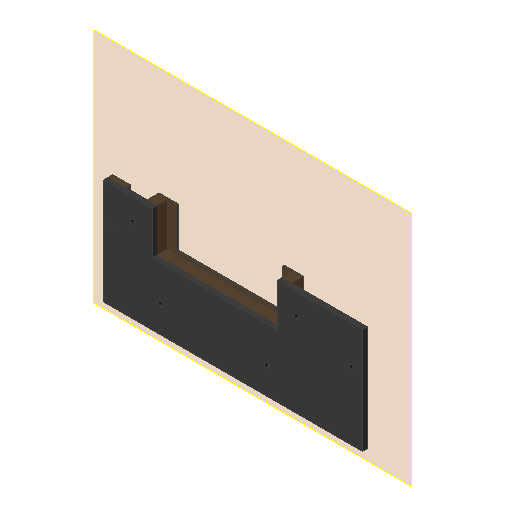
# Autodesk Inventor part: 30_XYTabel_Aliexpress_cellSTORM_chiptray
Saved by Autodesk Inventor 2022 (Build 260153000, 153)
## iProperties
Created: 2021-12-30
Part Number: 30_XYTabel_Aliexpress_cellSTORM_chiptray
Material: Generisch
Document SubType Name: Modeling
Designer: diederichbenedict
Density: 1 g/cm^3
Appearance: Vorgabe
Author: diederichbenedict
Autodesk Inventor part; units mm, degrees
ref_plane "YZ Plane" through (0, 0, 0) normal (1, 0, 0) x (0, 1, 0)
ref_plane "Arbeitsebene1" through (0, 0, 0) normal (0, 0, 1) x (1, 0, 0)
sketch "Skizze1" plane through (0, 0, 0) normal (0, 0, 1) x (1, 0, 0)
  circle A0 centre (-54.34, -50.59) radius 1.5 projected
  circle A1 centre (11.66, -50.59) radius 1.5 projected
  circle A2 centre (-85.34, -22.83) radius 1 projected
  circle A3 centre (-85.34, -22.83) radius 1 construction
  circle A4 centre (-85.34, 37.77) radius 1 construction
  line L0 (37.14, -42.13) -> (37.14, -36.73) construction
  arc A5 (32.14, -41.73) -> (37.14, -36.73) centre (32.14, -36.73) ccw construction
  line L1 (32.14, -41.73) -> (-73.22, -41.73) construction
  arc A6 (-78.22, -36.73) -> (-73.22, -41.73) centre (-73.22, -36.73) ccw construction
  line L2 (-78.22, -36.73) -> (-78.22, 48.27) construction
  arc A7 (-73.22, 53.27) -> (-78.22, 48.27) centre (-73.22, 48.27) ccw construction
  line L3 (-73.22, 53.27) -> (32.14, 53.27) construction
  arc A8 (37.14, 48.27) -> (32.14, 53.27) centre (32.14, 48.27) ccw construction
  line L4 (37.14, 48.27) -> (37.14, 54.21) construction
  line L5 (37.14, 54.21) -> (-89.84, 54.21) construction
  line L6 (-89.84, 54.21) -> (-89.84, -42.13) construction
  line L7 (-89.84, -42.13) -> (37.14, -42.13) construction
  circle A9 centre (64.84, -24.91) radius 1.5 construction
  circle A10 centre (-85.34, -43.41) radius 1 construction
  circle A11 centre (64.84, 35.59) radius 1.5 construction
  circle A12 centre (11.66, -50.59) radius 1.5 construction
  circle A13 centre (-54.34, -50.59) radius 1.5 construction
  circle A14 centre (-85.34, 58.59) radius 1 construction
  line L8 (-89.84, 67.09) -> (-89.84, 54.21) construction
  line L9 (-89.84, 54.21) -> (37.14, 54.21) construction
  line L10 (37.14, 54.21) -> (37.14, -42.13) construction
  line L11 (37.14, -42.13) -> (-89.84, -42.13) construction
  line L12 (-89.84, -42.13) -> (-89.84, -67.09) construction
  line L13 (-89.84, -67.09) -> (89.84, -67.09) construction
  line L14 (89.84, -67.09) -> (89.84, 67.09) construction
  line L15 (89.84, 67.09) -> (-89.84, 67.09) construction
  line L16 (-58.54, -1.33) -> (17.46, -1.33) construction
  line L17 (-58.54, -27.13) -> (-58.54, -1.33) construction
  line L18 (17.46, -27.13) -> (-58.54, -27.13) construction
  line L19 (17.46, -1.33) -> (17.46, -27.13) construction
  line L20 (-89.84, -1.33) -> (-59.54, -1.33)
  line L21 (-59.54, -1.33) -> (-59.54, -28.13)
  line L22 (-59.54, -28.13) -> (18.46, -28.13)
  line L23 (18.46, -28.13) -> (18.46, -1.33)
  line L24 (18.46, -1.33) -> (71.6268, -1.33)
  line L25 (71.6268, -1.33) -> (71.6268, -67.09)
  line L26 (71.6268, -67.09) -> (-89.84, -67.09)
  line L27 (-89.84, -1.33) -> (-89.84, -67.09)
  circle A15 centre (-54.34, -50.59) radius 1.5
  circle A16 centre (11.66, -50.59) radius 1.5
  circle A17 centre (-85.34, -22.83) radius 1
  circle A18 centre (64.84, -24.91) radius 1.5
  point P0 (0, 0)
  dimension "d0" = 1
  dimension "d1" = 1
  dimension "d2" = 1
  constraints: 16 end point, 6 perpendicular, 4 centre point, 4 coincident, 4 concentric, 4 point on line, 1 horizontal
  measures "d0" distance between parallel lines of L19 L23
  measures "d1" distance between parallel lines of L18 L22
  measures "d2" distance between parallel lines of L21 L17
extrude "Extrusion1" add sketch "Skizze1" along normal blind 3
sketch "Skizze2" plane through (0, 0, 0) normal (0, 0, -1) x (-1, 0, 0)
  circle A0 centre (85.34, -22.83) radius 1 projected
  circle A1 centre (85.34, 37.77) radius 1 projected
  line L0 (-37.14, -42.13) -> (-37.14, -36.73) projected
  arc A2 (-37.14, -36.73) -> (-32.14, -41.73) centre (-32.14, -36.73) ccw projected
  line L1 (-32.14, -41.73) -> (73.22, -41.73) projected
  arc A3 (73.22, -41.73) -> (78.22, -36.73) centre (73.22, -36.73) ccw projected
  line L2 (78.22, -36.73) -> (78.22, 48.27) projected
  arc A4 (78.22, 48.27) -> (73.22, 53.27) centre (73.22, 48.27) ccw projected
  line L3 (73.22, 53.27) -> (-32.14, 53.27) projected
  arc A5 (-32.14, 53.27) -> (-37.14, 48.27) centre (-32.14, 48.27) ccw projected
  line L4 (-37.14, 48.27) -> (-37.14, 54.21) projected
  line L5 (-37.14, 54.21) -> (89.84, 54.21) projected
  line L6 (89.84, 54.21) -> (89.84, -42.13) projected
  line L7 (89.84, -42.13) -> (-37.14, -42.13) projected
  line L8 (78.22, -36.73) -> (89.84, -36.73)
  line L9 (89.84, -1.33) -> (89.84, -67.09) projected
  line L10 (59.54, -1.33) -> (89.84, -1.33) projected
  line L11 (89.84, -36.73) -> (78.8105, -36.73)
  line L12 (78.8105, -36.73) -> (78.8105, -1.33)
  line L13 (78.8105, -1.33) -> (89.84, -1.33)
  line L14 (89.84, -1.33) -> (89.84, -36.73)
  point P0 (0, 0)
  constraints: 10 end point, 2 parallel, 2 perpendicular, 2 point on line, 1 horizontal
ref_plane "Arbeitsebene2" through (-89.84, -42.13, -2.77) normal (0, 0, 1) x (1, 0, 0)
extrude "Extrusion2" add sketch "Skizze2" along normal up to surface (2.77 mm away) contours L8 L12 L10 L6
ref_plane "Arbeitsebene3" through (-58.54, -27.13, -6.3955) normal (0, 0, -1) x (0, 1, 0)
sketch "Skizze3" plane through (0, 0, 0) normal (0, 0, -1) x (-1, 0, 0)
  line L0 (78.8105, -36.73) -> (78.8105, -1.33) projected
  line L1 (59.54, -1.33) -> (78.8105, -1.33) projected
  line L2 (59.54, -28.13) -> (59.54, -1.33) projected
  line L3 (-18.46, -28.13) -> (59.54, -28.13) projected
  line L4 (-18.46, -1.33) -> (-18.46, -28.13) projected
  line L5 (-71.6268, -1.33) -> (-18.46, -1.33) projected
  line L6 (-71.6268, -67.09) -> (-71.6268, -1.33) projected
  line L7 (89.84, -67.09) -> (-71.6268, -67.09) projected
  line L8 (89.84, -36.73) -> (89.84, -67.09) projected
  line L9 (89.84, -36.73) -> (78.8105, -36.73) projected
  circle A0 centre (-64.84, -24.91) radius 1.5 projected
  circle A1 centre (-11.66, -50.59) radius 1.5 projected
  circle A2 centre (54.34, -50.59) radius 1.5 projected
  line L10 (-18.46, -1.33) -> (-18.46, -28.13) projected
  line L11 (-18.46, -1.33) -> (-24.46, -1.33)
  line L12 (-24.46, -1.33) -> (-24.46, -28.13)
  line L13 (-24.46, -28.13) -> (-18.46, -28.13)
  line L14 (-18.46, -28.13) -> (-18.46, -1.33)
  line L15 (59.54, -1.33) -> (65.54, -1.33)
  line L16 (65.54, -1.33) -> (65.54, -28.13)
  line L17 (65.54, -28.13) -> (59.54, -28.13)
  line L18 (59.54, -28.13) -> (59.54, -1.33)
  line L19 (65.54, -28.13) -> (-24.46, -28.13)
  line L20 (-24.46, -28.13) -> (-24.46, -30.13)
  line L21 (-24.46, -30.13) -> (65.54, -30.13)
  line L22 (65.54, -30.13) -> (65.54, -28.13)
  point P0 (0, 0)
  dimension "d7" = 6
  dimension "d8" = 6
  dimension "d9" = 2
  constraints: 24 end point, 6 parallel, 3 horizontal, 3 perpendicular, 2 point on line
  measures "d7" distance of L13.end L12.end
  measures "d8" distance of L16.end L17.end
  measures "d9" distance of L20.end L19.end
extrude "Extrusion3" add sketch "Skizze3" along normal up to surface (6.3955 mm away) contours L16 L17 L2 L1 | L22 L21 L20 L13 L3 L17 | L13 L12 L5 L4
sketch "Skizze4" plane through (0, 0, -6.3955) normal (0, 0, -1) x (-1, 0, 0)
  line L0 (-18.46, -1.33) -> (-24.46, -1.33) projected
  line L1 (-24.46, -1.33) -> (-24.46, -30.13) projected
  line L2 (-24.46, -30.13) -> (65.54, -30.13) projected
  line L3 (65.54, -30.13) -> (65.54, -1.33) projected
  line L4 (65.54, -1.33) -> (59.54, -1.33) projected
  line L5 (59.54, -1.33) -> (59.54, -28.13) projected
  line L6 (59.54, -28.13) -> (-18.46, -28.13) projected
  line L7 (-18.46, -28.13) -> (-18.46, -1.33) projected
  line L8 (59.54, -1.33) -> (53.54, -1.33)
  line L9 (53.54, -1.33) -> (53.54, -28.13)
  line L10 (53.54, -28.13) -> (59.54, -28.13)
  line L11 (59.54, -28.13) -> (59.54, -1.33)
  line L12 (-18.46, -28.13) -> (59.54, -28.13) projected
  line L13 (-18.46, -28.13) -> (-12.46, -28.13)
  line L14 (-12.46, -28.13) -> (-12.46, -1.33)
  line L15 (-12.46, -1.33) -> (-18.46, -1.33)
  line L16 (-18.46, -1.33) -> (-18.46, -28.13)
  line L17 (-12.46, -28.13) -> (53.54, -28.13)
  line L18 (53.54, -28.13) -> (53.54, -26.13)
  line L19 (53.54, -26.13) -> (-12.46, -26.13)
  line L20 (-12.46, -26.13) -> (-12.46, -28.13)
  point P0 (0, 0)
  point P1 (-12.46, -26.13)
  dimension "d12" = 6
  dimension "d13" = 6
  dimension "d14" = 2
  constraints: 24 end point, 6 parallel, 3 horizontal, 3 perpendicular, 3 point on line
  measures "d12" distance of L10.end L9.end
  measures "d13" distance of L15.end L14.end
  measures "d14" distance of L18.end L17.end
extrude "Extrusion4" add sketch "Skizze4" along normal blind 1
sketch "Skizze5" plane through (0, 0, 3) normal (0, 0, 1) x (1, 0, 0)
  line L0 (-89.84, -67.09) -> (71.6268, -67.09) projected
  line L1 (71.6268, -67.09) -> (71.6268, -1.33) projected
  line L2 (71.6268, -1.33) -> (18.46, -1.33) projected
  line L3 (18.46, -1.33) -> (18.46, -28.13) projected
  line L4 (18.46, -28.13) -> (-59.54, -28.13) projected
  line L5 (-59.54, -28.13) -> (-59.54, -1.33) projected
  line L6 (-59.54, -1.33) -> (-89.84, -1.33) projected
  line L7 (-89.84, -1.33) -> (-89.84, -67.09) projected
  circle A0 centre (64.84, -24.91) radius 1.5 projected
  circle A1 centre (-85.34, -22.83) radius 1 projected
  circle A2 centre (11.66, -50.59) radius 1.5 projected
  circle A3 centre (-54.34, -50.59) radius 1.5 projected
  circle A4 centre (-71.54, -14.73) radius 1.4
  circle A5 centre (30.46, -14.73) radius 1.4
  point P0 (0, 0)
  dimension "d18" = 2.8
  dimension "d19" = 2.8
  dimension "d20" = 12
  dimension "d21" = 12
  constraints: 2 centre point
  measures "d18" diameter of A4
  measures "d19" diameter of A5
  measures "d20" distance from line of A4.centre L5
  measures "d21" distance from line of A5.centre L3
extrude "Extrusion5" cut sketch "Skizze5" against normal through all contours A4 | A5
